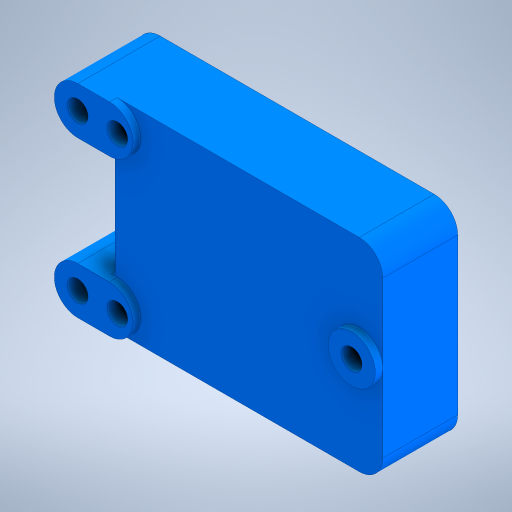
# Autodesk Inventor part: Lord Microstrain 3DM-CX5 OEM
Saved by Autodesk Inventor 2023 (Build 270158000, 158)
## iProperties
Created: 2022-07-03
Part Number: Lord Microstrain 3DM-CX5 OEM
Material: Generic
Document SubType Name: Modeling
Designer: Jochen Alt
Density: 1 g/cm^3
Appearance: Default
Author: Jochen Alt
Autodesk Inventor part; units mm, degrees
ref_plane "YZ Plane" through (0, 0, 0) normal (1, 0, 0) x (0, 1, 0)
ref_plane "XZ Plane" through (0, 0, 0) normal (0, 1, 0) x (-1, 0, 0)
ref_plane "XY Plane" through (0, 0, 0) normal (0, 0, 1) x (1, 0, 0)
sketch "Sketch1" plane through (0, 0, 0) normal (0, 0, 1) x (1, 0, 0)
  line L0 (-27.4801, 0) -> (27.4801, 0) construction
  line L1 (0, -17.6656) -> (0, 17.6656) construction
  line L2 (-16.256, 12.0396) -> (16.256, 12.0396)
  line L3 (19.05, 9.2456) -> (19.05, -9.2456)
  line L4 (16.256, -12.0396) -> (-16.256, -12.0396)
  line L5 (-19.05, -9.2456) -> (-19.05, 9.2456)
  line L6 (-16.256, 9.2456) -> (-16.256, -9.2456) construction
  circle A0 centre (-16.256, 9.2456) radius 1.2192
  circle A1 centre (-16.256, -9.2456) radius 1.2192
  circle A2 centre (16.256, 0) radius 1.2192
  arc A3 (-16.256, 12.0396) -> (-19.05, 9.2456) centre (-16.256, 9.2456) ccw
  arc A4 (-19.05, -9.2456) -> (-16.256, -12.0396) centre (-16.256, -9.2456) ccw
  arc A5 (16.256, -12.0396) -> (19.05, -9.2456) centre (16.256, -9.2456) ccw
  arc A6 (19.05, 9.2456) -> (16.256, 12.0396) centre (16.256, 9.2456) ccw
  line L7 (-16.256, 9.2456) -> (-12.4968, 9.2456) construction
  line L8 (-12.4968, 6.4516) -> (-16.256, 6.4516)
  arc A7 (-16.256, 12.0396) -> (-16.256, 6.4516) centre (-16.256, 9.2456) ccw
  arc A8 (-12.4968, 6.4516) -> (-12.4968, 12.0396) centre (-12.4968, 9.2456) ccw
  line L9 (-16.256, -9.2456) -> (-12.4968, -9.2456) construction
  line L10 (-12.4968, -6.4516) -> (-16.256, -6.4516)
  arc A9 (-16.256, -6.4516) -> (-19.05, -9.2456) centre (-16.256, -9.2456) ccw
  arc A10 (-12.4968, -12.0396) -> (-12.4968, -6.4516) centre (-12.4968, -9.2456) ccw
  circle A11 centre (-11.556, 9.2456) radius 1.2192
  circle A12 centre (-11.556, -9.2456) radius 1.2192
  line L11 (-11.556, 9.2456) -> (-11.556, -9.2456) construction
  line L12 (-12.7, 5.9436) -> (-12.7, -5.9436)
  arc A13 (-12.7, 5.9436) -> (-13.208, 6.4516) centre (-13.208, 5.9436) ccw
  arc A14 (-13.208, -6.4516) -> (-12.7, -5.9436) centre (-13.208, -5.9436) ccw
  circle A15 centre (16.256, 0) radius 2.794
  point P0 (0, 0)
  point P1 (19.05, -12.0396)
  point P2 (19.05, 12.0396)
  point P3 (-19.05, -12.0396)
  point P4 (-14.3764, 9.2456)
  point P5 (-14.3764, -9.2456)
  dimension "d0" = 38.1
  dimension "d1" = 24.0792
  dimension "d2" = 18.4912
  dimension "d3" = 2.4384
  dimension "d4" = 32.512
  dimension "d7" = 3.7592
  dimension "d8" = 4.7
  dimension "d9" = 6.35
  dimension "d12" = 0.508
  constraints: 26 end point, 21 tangent, 20 point on circle, 16 centre point, 15 point on line, 8 equal radius, 5 perpendicular, 4 coincident, 3 parallel, 2 midpoint, 1 horizontal, 1 vertical, 3 other
  measures "d0" distance of point (19.05, -12.04) point (-19.05, -12.04)
  measures "d1" distance of point (19.05, 12.04) point (19.05, -12.04)
  measures "d2" distance of L6.start L6.end
  measures "d3" diameter of A0
  measures "d4" distance from line of A2.centre L6
  measures "d7" distance of L7.end L6.start
  measures "d8" distance of L11.start L6.start
  measures "d9" distance between parallel lines of L12 L5
  measures "d12" radius of A13
extrude "Extrusion1" add sketch "Sketch1" along normal blind 1.905 contours L2 A8 L8 A7 A3 | A15 | L2 A6 L3 A5 L4 A10 L10 A14 L12 A13 L8 A8 | A7 L8 A13 L12 A14 L10 A9 L5 | A9 L10 A10 L4 A4 | A11 | A12
extrude "Extrusion2" add sketch "Sketch1" along normal blind 6.985 from surface at 1.905 contours L2 A8 L8 A7 A3 | A15 | L2 A6 L3 A5 L4 A10 L10 A14 L12 A13 L8 A8 | A9 L10 A10 L4 A4
extrude "Extrusion3" add sketch "Sketch1" along normal blind 0.889 from surface at 8.89 contours L2 A8 L8 A7 A3 | A15 | A9 L10 A10 L4 A4
body "Solid1"
